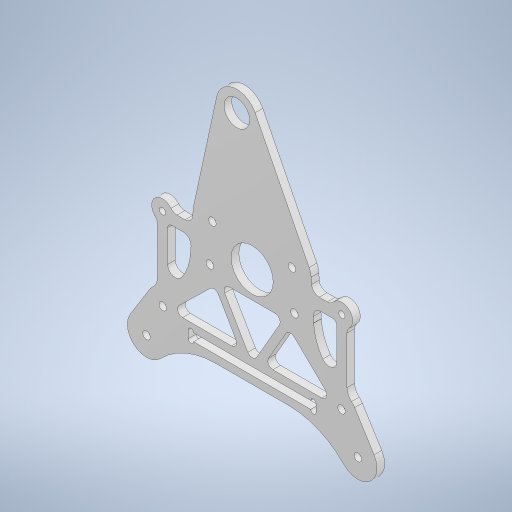
# Autodesk Inventor part: 中間ユニット内
Saved by Autodesk Inventor 2023 (Build 270158000, 158)
## iProperties
Created: 2022-03-07
Part Number: 中間ユニット内
Material: Aluminum 2014-T6
Document SubType Name: Modeling
Designer: acps
Density: 2.78927 g/cm^3
Appearance: Satin
Author: acps
Autodesk Inventor part; units mm, degrees
ref_plane "YZ Plane" through (0, 0, 0) normal (1, 0, 0) x (0, 1, 0)
ref_plane "XZ Plane" through (0, 0, 0) normal (0, 1, 0) x (-1, 0, 0)
ref_plane "XY Plane" through (0, 0, 0) normal (0, 0, 1) x (1, 0, 0)
sketch "Sketch2" plane through (0, 0, 0) normal (0, 0, 1) x (1, 0, 0)
  line L0 (0, 0) -> (0, 5.2095) construction
  circle A0 centre (0, 29.7999) radius 10.2397 construction
  arc A1 (-8.9837, 19.5602) -> (-10.7158, 16.5602) centre (-8.9837, 17.5602) ccw
  line L1 (-8.9837, 19.5602) -> (8.9837, 19.5602)
  arc A2 (10.7158, 16.5602) -> (8.9837, 19.5602) centre (8.9837, 17.5602) ccw
  line L2 (-10.7158, 16.5602) -> (-1.7321, 1)
  line L3 (10.7158, 16.5602) -> (1.7321, 1)
  arc A3 (-1.7321, 1) -> (1.7321, 1) centre (0, 2) ccw
  line L4 (-25, -4.5) -> (25, -4.5) construction
  line L5 (-23.95, -3) -> (-23.95, -6) construction
  line L6 (-25, -3) -> (-25, -6)
  line L7 (-22.9, -6) -> (-22.9, -3) construction
  arc A4 (-22.9, -3) -> (-25, -3) centre (-23.95, -3) ccw
  arc A5 (-25, -6) -> (-22.9, -6) centre (-23.95, -6) ccw
  arc A6 (25, -3) -> (22.9, -3) centre (23.95, -3) ccw
  line L8 (25, -3) -> (25, -6)
  arc A7 (22.9, -6) -> (25, -6) centre (23.95, -6) ccw
  line L9 (16.3793, 15.3817) -> (28.6251, 3.4314)
  arc A8 (27.2282, 0) -> (28.6251, 3.4314) centre (27.2282, 2) ccw
  line L10 (27.2282, 0) -> (8.0829, 0)
  line L11 (-25, -3) -> (-23.95, -3) construction
  line L12 (-22.9, -3) -> (22.9, -3)
  line L13 (-25, -6) -> (-23.95, -6) construction
  line L14 (-22.9, -6) -> (22.9, -6)
  line L15 (-26.5636, -1.95) -> (-22.5758, -1.95) construction
  line L16 (14.2621, -9) -> (0, -9)
  line L17 (-16.3793, 15.3817) -> (-28.6251, 3.4314)
  line L18 (-27.2282, 0) -> (-8.0829, 0)
  arc A9 (-28.6251, 3.4314) -> (-27.2282, 0) centre (-27.2282, 2) ccw
  line L19 (-14.2621, -9) -> (0, -9)
  arc A10 (16.3793, 15.3817) -> (13.2504, 14.9503) centre (14.9824, 13.9503) ccw
  line L20 (13.2504, 14.9503) -> (6.3509, 3)
  arc A11 (6.3509, 3) -> (8.0829, 0) centre (8.0829, 2) ccw
  arc A12 (-13.2504, 14.9503) -> (-16.3793, 15.3817) centre (-14.9824, 13.9503) ccw
  line L21 (-13.2504, 14.9503) -> (-6.3509, 3)
  arc A13 (-8.0829, 0) -> (-6.3509, 3) centre (-8.0829, 2) ccw
  circle A14 centre (16.5506, 23.3453) radius 7.525
  circle A15 centre (15.5646, 38.363) radius 7.525
  line L22 (34.0353, 7.514) -> (38.0125, 5.2178)
  circle A16 centre (41.3199, -13) radius 7.525
  line L23 (15.5646, 45.888) -> (7.3682, 45.888)
  line L24 (-15.5646, 45.888) -> (7.3682, 45.888)
  line L25 (-14.2621, -9) -> (0, -9)
  circle A17 centre (35, 0) radius 1.5
  circle A18 centre (35, 0) radius 3.025
  circle A19 centre (35, 0) radius 6.025
  circle A20 centre (-35, 0) radius 6.025
  circle A21 centre (-35, 0) radius 3.025
  circle A22 centre (-35, 0) radius 1.5
  circle A23 centre (16.5506, 23.3453) radius 3.025
  circle A24 centre (41.3199, -13) radius 3.025
  line L26 (47.7096, -9.0254) -> (40.116, 3.1823)
  line L27 (-20.812, -60) -> (26.178, -60)
  circle A25 centre (-6, 80) radius 5.025
  circle A26 centre (-6, 80) radius 8.025
  arc A27 (35.8939, -18.2139) -> (14.2621, -9) centre (14.2621, -39) ccw
  circle A28 centre (0, 29.7999) radius 8.2397
  arc A29 (26.1288, 47.4363) -> (20.0049, 23.2712) centre (35.6549, 32.1637) ccw construction
  line L28 (22.3769, 18.583) -> (19.6218, 23.982) construction
  arc A30 (61.1577, -34.4951) -> (56.1103, -14.552) centre (52.6424, -26.04) ccw construction
  arc A31 (61.1577, -34.4951) -> (60.8311, -36.8802) centre (62.5769, -35.9043) ccw construction
  arc A32 (60.8311, -36.8802) -> (78.0598, -53.6221) centre (97.4928, -16.3882) ccw construction
  arc A33 (53.2941, -13.5379) -> (56.1103, -14.552) centre (64.3583, 12.7718) ccw construction
  arc A34 (26.0209, 0.9091) -> (22.8953, 17.5672) centre (-3.8265, 3.9311) ccw construction
  arc A35 (53.2941, -13.5379) -> (34.3508, -9.0016) centre (30.0348, -68.8462) ccw construction
  circle A36 centre (15.5646, 38.363) radius 1.5
  circle A37 centre (15.5646, 38.363) radius 3.025
  line L29 (23.0735, 38.856) -> (24.0594, 23.8383)
  circle A38 centre (16.5506, 23.3453) radius 1.5
  circle A39 centre (41.3199, -13) radius 1.5
  circle A40 centre (-41.3199, -13) radius 7.525
  circle A41 centre (-41.3199, -13) radius 3.025
  circle A42 centre (-41.3199, -13) radius 1.5
  circle A43 centre (-35, 0) radius 6.025
  circle A44 centre (-35, 0) radius 3.025
  circle A45 centre (-35, 0) radius 1.5
  circle A46 centre (-16.5506, 23.3453) radius 7.525
  circle A47 centre (-16.5506, 23.3453) radius 1.5
  circle A48 centre (-16.5506, 23.3453) radius 3.025
  circle A49 centre (-15.5646, 38.363) radius 7.525
  circle A50 centre (-15.5646, 38.363) radius 3.025
  circle A51 centre (-15.5646, 38.363) radius 1.5
  arc A52 (-14.2621, -9) -> (-35.8939, -18.2139) centre (-14.2621, -39) ccw
  line L30 (-47.7096, -9.0254) -> (-40.116, 3.1823)
  line L31 (-34.0353, 7.514) -> (-38.0125, 5.2178)
  line L32 (-23.0735, 38.856) -> (-24.0594, 23.8383)
  arc A53 (24.0646, 23.7525) -> (34.0353, 7.514) centre (44.0353, 24.8346) ccw
  arc A54 (-34.0353, 7.514) -> (-24.0646, 23.7525) centre (-44.0353, 24.8346) ccw
  circle A55 centre (35.0898, 32.1644) radius 1.25
  circle A56 centre (35.0898, 32.1644) radius 4.25
  line L33 (35.0898, 32.1644) -> (22.0882, 32.1644) construction
  line L34 (29.4054, 33.6644) -> (26.2238, 33.6644)
  arc A57 (29.4054, 33.6644) -> (31.7576, 34.8023) centre (29.4054, 36.6644) ccw
  arc A58 (23.2303, 36.4678) -> (26.2238, 33.6644) centre (26.2238, 36.6644) ccw
  line L35 (26.9132, 29.1644) -> (31.4681, 29.1644)
  line L36 (35.0898, 32.1644) -> (35.0898, 8.7801) construction
  arc A59 (33.0898, 27.5427) -> (31.4681, 29.1644) centre (31.4681, 27.5427) ccw
  line L37 (33.0898, 27.5427) -> (33.0898, 15.1122)
  arc A60 (26.9132, 29.1644) -> (23.9196, 25.9678) centre (26.9132, 26.1644) ccw
  arc A61 (27.6288, 13.3965) -> (33.0898, 15.1122) centre (30.0898, 15.1122) ccw
  line L38 (37.0898, 26.9144) -> (37.0898, 8.4431)
  arc A62 (37.0898, 8.4431) -> (38.8745, 4.614) centre (42.0898, 8.4431) ccw
  arc A63 (38.0208, 29.0868) -> (37.0898, 26.9144) centre (40.0898, 26.9144) ccw
  arc A64 (-38.8745, 4.614) -> (-37.0898, 8.4431) centre (-42.0898, 8.4431) ccw
  line L39 (-37.0898, 26.9144) -> (-37.0898, 8.4431)
  arc A65 (-33.0898, 15.1122) -> (-27.6288, 13.3965) centre (-30.0898, 15.1122) ccw
  line L40 (-33.0898, 27.5427) -> (-33.0898, 15.1122)
  circle A66 centre (-35.0898, 32.1644) radius 4.25
  arc A67 (-37.0898, 26.9144) -> (-38.0208, 29.0868) centre (-40.0898, 26.9144) ccw
  arc A68 (-31.4681, 29.1644) -> (-33.0898, 27.5427) centre (-31.4681, 27.5427) ccw
  line L41 (-26.9132, 29.1644) -> (-31.4681, 29.1644)
  arc A69 (-23.9196, 25.9678) -> (-26.9132, 29.1644) centre (-26.9132, 26.1644) ccw
  arc A70 (-26.2238, 33.6644) -> (-23.2303, 36.4678) centre (-26.2238, 36.6644) ccw
  line L42 (-29.4054, 33.6644) -> (-26.2238, 33.6644)
  arc A71 (-31.7576, 34.8023) -> (-29.4054, 33.6644) centre (-29.4054, 36.6644) ccw
  circle A72 centre (-35.0898, 32.1644) radius 1.25
  line L43 (-13.8418, 81.705) -> (-22.9178, 39.9618)
  line L44 (1.1649, 83.6145) -> (22.2831, 41.7523)
  point P0 (-23.95, -4.5)
  point P1 (0, 0)
  point P2 (-38.8745, 4.614)
  point P3 (-40.116, 3.1823)
  point P4 (-35.8939, -18.2139)
  point P5 (-27.6288, 13.3965)
  dimension "d361" = 2
  dimension "d362" = 2
  dimension "d363" = 30
  dimension "d364" = 2
  dimension "d365" = 50
  dimension "d366" = 3
  dimension "d367" = 2.1
  dimension "d368" = 25
  dimension "d369" = 2
  dimension "d370" = 60
  dimension "d371" = 3
  dimension "d372" = 2
  dimension "d373" = 2
  dimension "d374" = 3
  dimension "d375" = 3
  dimension "d376" = 6.05
  dimension "d377" = 3
  dimension "d378" = 30
  dimension "d379" = 6.05
  dimension "d380" = 6.05
  dimension "d381" = 60
  dimension "d382" = 10.05
  dimension "d383" = 3
  dimension "d384" = 4.5
  dimension "d385" = 30
  dimension "d386" = 2
  dimension "d387" = 3
  dimension "d388" = 6.05
  dimension "d389" = 4.5
  dimension "d390" = 4.5
  dimension "d391" = 4.5
  dimension "d392" = 13
  dimension "d393" = 3
  dimension "d394" = 3
  dimension "d395" = 20
  dimension "d396" = 6
  dimension "d397" = 80
  dimension "d398" = 2.5
  dimension "d399" = 3
  dimension "d400" = 1.5
  dimension "d401" = 3
  dimension "d402" = 3
  dimension "d403" = 2
  dimension "d404" = 3
  dimension "d405" = 3
  dimension "d406" = 3
  dimension "d407" = 5
  dimension "d408" = 2
  dimension "d409" = 3
  constraints: 96 point on circle, 92 end point, 72 centre point, 62 symmetric about line, 54 tangent, 18 coincident, 10 horizontal, 7 parallel, 4 point on line, 4 vertical, 3 midpoint, 1 equal radius, 1 horizontal alignment, 1 vertical alignment, 47 other
  measures "d361" radius of A2
  measures "d362" radius of A3
  measures "d363" angle of L0 L2
  measures "d364" radius of A1
  measures "d365" distance of L4.start L4.end
  measures "d366" distance of L5.start L5.end
  measures "d367" diameter of A5
  measures "d368" horizontal distance of point (-25, -4.5) L0.start
  measures "d369" radius of A8
  measures "d370" angle of L2 L3
  measures "d371" distance between parallel lines of L16 L14
  measures "d372" radius of A10
  measures "d373" radius of A11
  measures "d374" distance between parallel lines of L3 L20
  measures "d375" diameter of A17
  measures "d376" diameter of A18
  measures "d377" radial gap between concentric circles of A18 A19
  measures "d378" angle of L10 L22
  measures "d379" diameter of A23
  measures "d380" diameter of A24
  measures "d381" distance from line of point (0, 0) L27
  measures "d382" diameter of A25
  measures "d383" radial gap between concentric circles of A25 A26
  measures "d384" distance from line of L4 L0.start
  measures "d385" radius of A27
  measures "d386" radial gap between concentric circles of A28 A0
  measures "d387" diameter of A36
  measures "d388" diameter of A37
  measures "d389" radial gap between concentric circles of A16 A24
  measures "d390" radial gap between concentric circles of A14 A23
  measures "d391" radial gap between concentric circles of A15 A37
  measures "d392" distance from line of L10 A16.centre
  measures "d393" diameter of A38
  measures "d394" diameter of A39
  measures "d395" radius of A53
  measures "d396" horizontal distance of L0.start A25.centre
  measures "d397" vertical distance of L0.start A25.centre
  measures "d398" diameter of A55
  measures "d399" radial gap between concentric circles of A55 A56
  measures "d400" distance between parallel lines of L33 L34
  measures "d401" radius of A57
  measures "d402" radius of A58
  measures "d403" distance between parallel lines of L37 L36
  measures "d404" radius of A60
  measures "d405" distance between parallel lines of L33 L35
  measures "d406" radius of A61
  measures "d407" radius of A62
  measures "d408" distance between parallel lines of L36 L38
  measures "d409" radius of A63
extrude "Extrusion7" add sketch "Sketch2" against normal blind 3 contours A1 A46 A49 L24 L23 A15 A14 A2 L1 | A1 L2 A3 L3 A2 A14 A10 L20 A11 L10 A8 A19 L26 A16 A27 L16 L19 A52 A40 L30 A20 A9 L18 A13 L21 A12 A46 | A46 | A12 L17 A9 A20 L31 A54 A46 | A14 | A46 L32 A49 | A49 | A15 L29 A14 | A15 | A14 A53 L22 A19 A8 L9 A10 | A54 L31 A20 A64 L39 A67 A66 A68 L40 A65 | L23 L24 A49 L43 A26 L44 A15 | A20 | A69 L41 A68 A66 A71 L42 A70 L32 | L29 A58 L34 A57 A56 A59 L35 A60 | A26 | A61 L37 A59 A56 A63 L38 A62 A19 L22 A53 | A19 | A66 | A40 | A56 | A16
extrude "Extrusion8" add sketch "Sketch2" against normal blind 2 contours A18 | A21 | A23 | A24 | A37 | A41 | A48 | A50
body "Solid4"
